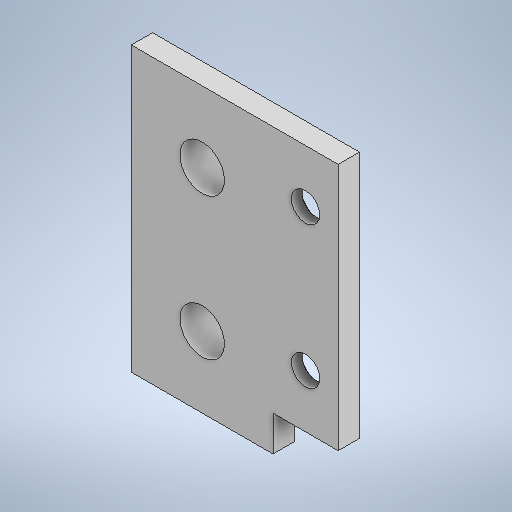
# Autodesk Inventor part: Base Rodamiento delgado
Saved by Autodesk Inventor 2025 (Build 290162000, 162)
## iProperties
Created: 2025-05-25
Part Number: Base Rodamiento delgado
Material: Genérico
Document SubType Name: Modeling
Designer: STEVEN LONDOÑO
Density: 1 g/cm^3
Appearance: Valor por defecto
Author: STEVEN LONDOÑO
Autodesk Inventor part; units mm, degrees
ref_plane "YZ Plane" through (0, 0, 0) normal (1, 0, 0) x (0, 1, 0)
ref_plane "XZ Plane" through (0, 0, 0) normal (0, 1, 0) x (-1, 0, 0)
ref_plane "XY Plane" through (0, 0, 0) normal (0, 0, 1) x (1, 0, 0)
sketch "Boceto1" plane through (0, 0, 0) normal (0, 0, 1) x (1, 0, 0)
  line L0 (-26.5284, 23.7303) -> (2.6646, 23.7303)
  line L1 (-6.5284, -16.2697) -> (-26.5284, -16.2697)
  line L2 (-26.5284, -16.2697) -> (-26.5284, 23.7303)
  line L3 (-26.5284, 23.7303) -> (-6.5284, 23.7303)
  line L4 (-6.5284, 23.7303) -> (-6.5284, -16.2697)
  line L5 (-6.5284, -16.2697) -> (-26.5284, -16.2697)
  line L6 (-26.5284, -16.2697) -> (-26.5284, 23.7303)
  circle A0 centre (-16.5284, 13.7303) radius 3.15
  circle A1 centre (-16.5284, -6.2697) radius 3.15
  circle A2 centre (-16.5284, -6.2697) radius 5.05
  circle A3 centre (-16.5284, 13.7303) radius 5.0326
  line L7 (-6.5284, 23.7303) -> (-1.9384, 23.7303)
  circle A4 centre (-1.9384, 16.2303) radius 2
  line L8 (-6.5284, 23.7303) -> (2.6646, 23.7303)
  line L9 (2.6646, 23.7303) -> (2.6646, -11.2697)
  line L10 (2.6646, -11.2697) -> (-6.5284, -11.2697)
  line L11 (-6.5284, -11.2697) -> (-6.5284, 23.7303)
  circle A5 centre (-1.9319, -3.7697) radius 2
  circle A6 centre (-1.9319, -3.7697) radius 4.05
  circle A7 centre (-1.9384, 16.2303) radius 4.05
  point P0 (0, 0)
  point P1 (13.9631, 1.0984)
  point P2 (-16.5284, 23.7303)
  dimension "d0" = 6.3
  dimension "d1" = 6.3
  dimension "d2" = 10
  dimension "d3" = 10
  dimension "d4" = 10.1
  dimension "d5" = 4.59
  dimension "d6" = 4
  dimension "d7" = 7.5
  dimension "d8" = 35
  dimension "d9" = 4
  dimension "d10" = 7.5
  dimension "d11" = 8.1
  dimension "d12" = 8.1
  constraints: 24 end point, 8 centre point, 5 parallel, 4 coincident, 3 horizontal, 2 perpendicular, 1 midpoint, 1 point on line
  measures "d0" diameter of A0
  measures "d1" diameter of A1
  measures "d2" distance of point (-16.528, 23.73) A0.centre
  measures "d3" distance from line of L1 A1.centre
  measures "d4" diameter of A2
  measures "d5" distance of L7.start L7.end
  measures "d6" diameter of A4
  measures "d7" distance from line of L0 A4.centre
  measures "d8" distance of L8.end L9.end
  measures "d9" diameter of A5
  measures "d10" distance from line of L10 A5.centre
  measures "d11" diameter of A6
  measures "d12" diameter of A7
extrude "Extrusión1" add sketch "Boceto1" along normal blind 3 contours L0 L4 L1 L2 | L0 L9 L10 L4
sketch "Boceto2" plane through (0, 0, 0) normal (0, 0, -1) x (-1, 0, 0)
  point P0 (0, 0)
sketch "Boceto3" plane through (0, 0, 3) normal (0, 0, 1) x (1, 0, 0)
  circle A0 centre (-1.9384, 16.2303) radius 4.05 projected
  circle A1 centre (-1.9384, 16.2303) radius 2
  circle A2 centre (-1.9319, -3.7697) radius 4.05 projected
  circle A3 centre (-1.9319, -3.7697) radius 2
  circle A4 centre (-16.5284, -6.2697) radius 5.05 projected
  circle A5 centre (-16.5284, -6.2697) radius 3.15
  circle A6 centre (-16.5284, 13.7303) radius 5.0326 projected
  circle A7 centre (-16.5284, 13.7303) radius 3.15
  point P0 (0, 0)
  dimension "d15" = 4
  dimension "d16" = 4
  dimension "d17" = 6.3
  dimension "d18" = 6.3
  constraints: 4 centre point, 4 coincident
  measures "d15" diameter of A1
  measures "d16" diameter of A3
  measures "d17" diameter of A5
  measures "d18" diameter of A7
extrude "Extrusión2" add sketch "Boceto3" against normal blind 1.5 contours A0 | A2
extrude "Extrusión3" add sketch "Boceto3" against normal blind 6 contours A4 | A6
